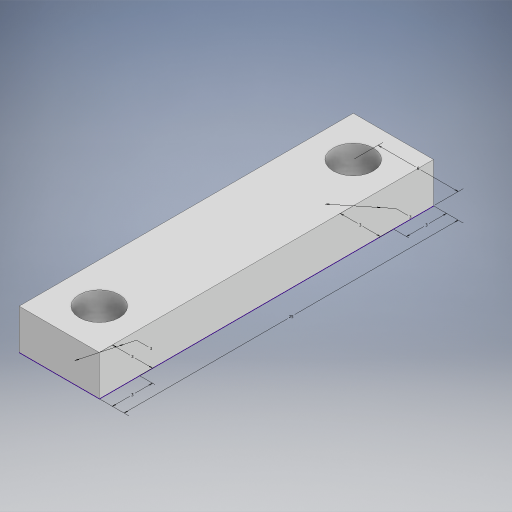
# Autodesk Inventor part: Akrilik Kabel SD Serayu
Saved by Autodesk Inventor 2024 (Build 280153000, 153)
## iProperties
Created: 2024-07-12
Part Number: Akrilik Kabel SD Serayu
Material: Generic
Document SubType Name: Modeling
Designer: LENOVO
Density: 1 g/cm^3
Appearance: Default
Author: LENOVO
Autodesk Inventor part; units mm, degrees
ref_plane "YZ Plane" through (0, 0, 0) normal (1, 0, 0) x (0, 1, 0)
ref_plane "XZ Plane" through (0, 0, 0) normal (0, 1, 0) x (-1, 0, 0)
ref_plane "XY Plane" through (0, 0, 0) normal (0, 0, 1) x (1, 0, 0)
sketch "Sketch1" plane through (0, 0, 0) normal (0, 1, 0) x (-1, 0, 0)
  line L0 (3, 12.5) -> (-3, 12.5)
  line L1 (-3, 12.5) -> (-3, -12.5)
  line L2 (-3, -12.5) -> (3, -12.5)
  line L3 (3, -12.5) -> (3, 12.5)
  line L4 (3, 12.5) -> (-3, -12.5) construction
  line L5 (-3, 12.5) -> (3, -12.5) construction
  line L6 (-3, -12.5) -> (-3, -9.5)
  line L7 (-3, -9.5) -> (0, -9.5)
  circle A0 centre (0, -9.5) radius 1.5
  line L8 (-3, 12.5) -> (-3, 9.5)
  line L9 (-3, 9.5) -> (0, 9.5)
  circle A1 centre (0, 9.5) radius 1.5
  point P0 (0, 0)
  dimension "d0" = 6
  dimension "d1" = 25
  dimension "d4" = 3
  dimension "d5" = 3
  dimension "d6" = 3
  dimension "d7" = 3
  dimension "d8" = 3
  dimension "d9" = 3
  constraints: 20 end point, 3 perpendicular, 2 centre point, 2 coincident, 2 midpoint, 2 parallel, 2 point on line, 1 horizontal
  measures "d0" distance of L2.end L1.end
  measures "d1" distance of L1.end L0.end
  measures "d4" distance of L1.end L6.end
  measures "d5" distance of L6.end L7.end
  measures "d6" diameter of A0
  measures "d7" distance of L0.end L8.end
  measures "d8" distance of L8.end L9.end
  measures "d9" diameter of A1
extrude "Extrusion1" add sketch "Sketch1" along normal blind 3 contours A1 | A0 | L3 L2 L1 L0
extrude "Extrusion2" cut sketch "Sketch1" along normal blind 3 contours A0
extrude "Extrusion3" cut sketch "Sketch1" along normal blind 3 contours A1
body "Solid1"
